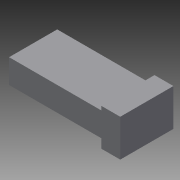
# Autodesk Inventor part: Resistant
Saved by Autodesk Inventor 2014 (Build 180170000, 170)
## iProperties
Created: 2014-04-24
Part Number: Resistant
Material: Generic
Document SubType Name: Modeling
Designer: Paul
Density: 1 g/cm^3
Appearance: Default
Author: Paul
Autodesk Inventor part; units mm, degrees
ref_plane "YZ Plane" through (0, 0, 0) normal (1, 0, 0) x (0, 1, 0)
ref_plane "XZ Plane" through (0, 0, 0) normal (0, 1, 0) x (-1, 0, 0)
ref_plane "XY Plane" through (0, 0, 0) normal (0, 0, 1) x (1, 0, 0)
sketch "Sketch1" plane through (0, 0, 0) normal (1, 0, 0) x (0, 1, 0)
  line L0 (-1.27, -2.54) -> (1.27, -2.54)
  line L1 (1.27, -2.54) -> (1.27, 2.54)
  line L2 (1.27, 2.54) -> (-1.27, 2.54)
  line L3 (-1.27, 2.54) -> (-1.27, -2.54)
  line L4 (-1.27, -2.54) -> (1.27, 2.54) construction
  line L5 (1.27, -2.54) -> (-1.27, 2.54) construction
  point P0 (0, 0)
  dimension "d2" = 2.54
  dimension "d3" = 5.08
  constraints: 12 end point, 2 midpoint, 2 parallel, 1 horizontal, 1 perpendicular
  measures "d2" distance of L1.end L2.end
  measures "d3" distance of L2.end L0.start
extrude "Extrusion1" add sketch "Sketch1" along normal blind 10
sketch "Sketch3" plane through (10, 0, 0) normal (1, 0, 0) x (0, 0, -1)
  line L0 (-2.809, 1.9578) -> (2.809, 1.9578)
  line L1 (2.809, 1.9578) -> (2.809, -1.9578)
  line L2 (2.809, -1.9578) -> (-2.809, -1.9578)
  line L3 (-2.809, -1.9578) -> (-2.809, 1.9578)
  line L4 (-2.809, 1.9578) -> (2.809, -1.9578) construction
  line L5 (2.809, 1.9578) -> (-2.809, -1.9578) construction
  point P0 (0, 0)
  constraints: 12 end point, 2 midpoint, 2 parallel, 1 horizontal, 1 perpendicular
extrude "Extrusion2" add sketch "Sketch3" along normal blind 2
body "Solid1"
